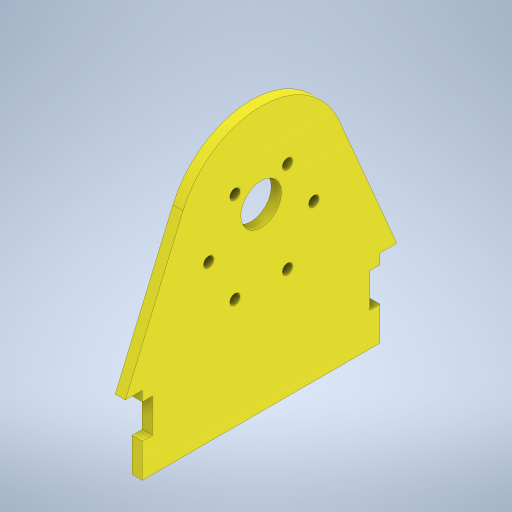
# Autodesk Inventor part: baseSoporte3
Saved by Autodesk Inventor 2024.3 (Build 283343000, 343)
## iProperties
Created: 2024-05-14
Part Number: baseSoporte3
Material: PMMA Plastic
Document SubType Name: Modeling
Designer: USUARIO
Density: 1.188 g/cm^3
Appearance: Canary
Mass: 15.1746 g
Surface Area: 94.6312 cm^2
Volume: 12.7732 cm^3
Author: USUARIO
Autodesk Inventor part; units mm, degrees
ref_plane "YZ Plane" through (0, 0, 0) normal (1, 0, 0) x (0, 1, 0)
ref_plane "XZ Plane" through (0, 0, 0) normal (0, 1, 0) x (-1, 0, 0)
ref_plane "XY Plane" through (0, 0, 0) normal (0, 0, 1) x (1, 0, 0)
sketch "Sketch1" plane through (0, 0, 0) normal (1, 0, 0) x (0, 1, 0)
  circle A0 centre (0, 0) radius 6
  line L0 (-30, -40) -> (9.8205, -22.9904)
  line L1 (-30, 40) -> (9.8205, 22.9904)
  line L2 (-33, -35) -> (-30, -35)
  line L3 (-33, 35) -> (-30, 35)
  line L4 (-46, 35) -> (-46, -35) construction
  line L5 (-30, 35) -> (-30, 40)
  line L6 (-30, -35) -> (-30, -40)
  line L7 (-43, 35) -> (-46, 35)
  arc A1 (9.8205, -22.9904) -> (9.8205, 22.9904) centre (0, 0) ccw
  circle A2 centre (6.4234, 7.75) radius 1.5
  circle A3 centre (6.4234, -7.75) radius 1.5
  circle A4 centre (-7, -15.5) radius 1.5
  circle A5 centre (-20.4234, -7.75) radius 1.5
  circle A6 centre (-20.4234, 7.75) radius 1.5
  circle A7 centre (-7, 15.5) radius 1.5
  line L8 (-46, -35) -> (-43, -35)
  line L9 (-43, -35) -> (-43, -32)
  line L10 (-43, -32) -> (-33, -32)
  line L11 (-33, -32) -> (-33, -35)
  line L12 (-43, 35) -> (-43, 32)
  line L13 (-43, 32) -> (-33, 32)
  line L14 (-33, 32) -> (-33, 35)
  line L15 (-46, 35) -> (-53, 35)
  line L16 (-53, 35) -> (-53, -35)
  line L17 (-53, -35) -> (-46, -35)
  point P0 (-46, 0)
  dimension "d0" = 12
  dimension "d40" = 70
  dimension "d58" = 25
  dimension "d59" = 5
  dimension "d61" = 39.8205
  dimension "d62" = 17.0096
  dimension "d63" = 39.8205
  dimension "d68" = 80
  dimension "d70" = 46
  dimension "d76" = 9.8205
  dimension "d79" = 3
  dimension "d80" = 3
  dimension "d81" = 3
  dimension "d82" = 3
  dimension "d83" = 3
  dimension "d84" = 3
  dimension "d89" = 7
  dimension "d90" = 7
  dimension "d91" = 15.5
  dimension "d92" = 15.5
  dimension "d93" = 7.75
  dimension "d94" = 7.75
  dimension "d95" = 20.4234
  dimension "d96" = 20.4234
  dimension "d97" = 7.75
  dimension "d98" = 7.75
  dimension "d99" = 6.4234
  dimension "d100" = 6.4234
  dimension "d105" = 3
  dimension "d108" = 3
  dimension "d112" = 3
  dimension "d113" = 5
  dimension "d116" = 3
  dimension "d117" = 3
  dimension "d118" = 10
  dimension "d119" = 3
  dimension "d120" = 3
  dimension "d121" = 10
  dimension "d122" = 3
  dimension "d123" = 7
  dimension "d124" = 70
  dimension "d125" = 7
  constraints: 36 end point, 8 centre point, 8 perpendicular, 3 horizontal, 2 coincident, 2 point on circle, 2 tangent, 2 vertical, 1 midpoint
  measures "d0" diameter of A0
  measures "d40" distance of L4.end L4.start
  measures "d58" radius of A1
  measures "d59" distance of L3.end L1.start
  measures "d61" distance from line of L1.end L5
  measures "d62" vertical distance of L1.end L1.start
  measures "d63" horizontal distance of L0.start L0.end
  measures "d68" distance of L0.start L1.start
  measures "d70" distance from line of L4 A1.centre
  measures "d76" horizontal distance of A1.centre L1.end
  measures "d79" diameter of A2
  measures "d80" diameter of A3
  measures "d81" diameter of A4
  measures "d82" diameter of A5
  measures "d83" diameter of A6
  measures "d84" diameter of A7
  measures "d89" horizontal distance of A7.centre A1.centre
  measures "d90" horizontal distance of A4.centre A1.centre
  measures "d91" vertical distance of A1.centre A4.centre
  measures "d92" vertical distance of A1.centre A7.centre
  measures "d93" vertical distance of A1.centre A6.centre
  measures "d94" vertical distance of A5.centre A1.centre
  measures "d95" horizontal distance of A1.centre A5.centre
  measures "d96" horizontal distance of A1.centre A6.centre
  measures "d97" vertical distance of A1.centre A2.centre
  measures "d98" vertical distance of A3.centre A1.centre
  measures "d99" horizontal distance of A1.centre A2.centre
  measures "d100" horizontal distance of A1.centre A3.centre
  measures "d105" distance of L7.start L4.start
  measures "d108" distance of L3.start L3.end
  measures "d112" distance of L2.start L2.end
  measures "d113" distance of L2.end L0.start
  measures "d116" distance of L4.end L8.end
  measures "d117" distance of L8.end L9.end
  measures "d118" distance of L9.end L10.end
  measures "d119" distance of L10.end L2.start
  measures "d120" distance of L7.start L12.end
  measures "d121" distance of L12.end L13.end
  measures "d122" distance of L13.end L3.start
  measures "d123" distance of L4.start L15.end
  measures "d124" distance of L15.end L16.end
  measures "d125" distance of L16.end L4.end
extrude "Extrusion1" add sketch "Sketch1" along normal blind 3
body "Solid1"
